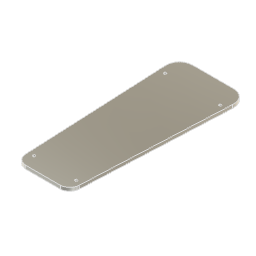
mission_engineering_pr1_pedal_raiser_kit v1 (Autodesk Fusion 360 design; units mm, degrees)
Autodesk Fusion 360 part; units mm, degrees
sketch "Sketch2" plane through (0, 0, 0) normal (0, 0, 1) x (1, 0, 0)
  line L0 (-41, 95) -> (40.1, 95) construction
  circle A0 centre (-41, 95) radius 1.75
  circle A1 centre (40.1, 95) radius 1.75
  line L1 (-32.1418, -106.2761) -> (29.9104, -106.2761) construction
  circle A2 centre (-32.1418, -106.2761) radius 1.75
  circle A3 centre (29.9104, -106.2761) radius 1.75
  line L2 (0, 125.7) -> (-30.2729, 125.7)
  line L3 (0, -124.4) -> (-26.7617, -124.4)
  line L4 (-40.5, -110.5) -> (-50.5, 104.7)
  arc A4 (-40.5, -110.5) -> (-26.7617, -124.4) centre (-25.9132, -109.8222) ccw
  arc A5 (-45.3008, 119.9335) -> (-50.5, 104.7) centre (-28.5694, 105.7191) ccw
  arc A6 (-30.2729, 125.7) -> (-45.3008, 119.9335) centre (-30.2729, 103.2348) ccw
  arc A7 (43.3008, 119.9335) -> (28.2729, 125.7) centre (28.2729, 103.2348) ccw
  arc A8 (48.5, 104.7) -> (43.3008, 119.9335) centre (26.5694, 105.7191) ccw
  line L5 (38.5, -110.5) -> (48.5, 104.7)
  arc A9 (24.7617, -124.4) -> (38.5, -110.5) centre (23.9132, -109.8222) ccw
  line L6 (0, 125.7) -> (28.2729, 125.7)
  line L7 (0, -124.4) -> (24.7617, -124.4)
  circle A10 centre (-41, 95) radius 3.75
  circle A11 centre (-41, 95) radius 3.75
  circle A12 centre (40.1, 95) radius 3.75
  circle A13 centre (-32.1418, -106.2761) radius 3.75
  circle A14 centre (29.9104, -106.2761) radius 3.75
  dimension "d1" = 3.5
  dimension "d2" = 62.0522
  dimension "d3" = 7.5
  dimension "d4" = 7.5
  constraint coincident L0.start A0.centre
  constraint coincident L0.end A1.centre
  constraint equal A0 A1
  constraint horizontal L1
  constraint coincident L1.start A2.centre
  constraint coincident L1.end A3.centre
  constraint equal A0 A2
  constraint equal A0 A3
  constraint tangent L4 A4
  constraint tangent L4 A5
  constraint tangent L2 A6
  constraint tangent A7 L6
  constraint parallel L3 L7
  constraint concentric A0 A10
  constraint concentric A1 A12
  constraint concentric A2 A13
  constraint concentric A3 A14
  constraint equal A10 A12
  constraint equal A10 A13
  constraint equal A10 A14
  measures "d1" diameter of A0
  measures "d2" distance of L1.start L1.end
  measures "d3" diameter of A10
  measures "d4" diameter of A11
extrude "Extrude1" add sketch "Sketch2" along normal blind 5 contours L2 L3 L4 A4 A5 A6 A7 A8 L5 A9 L6 L7 | A10 A11 | A12 | A13 | A14
extrude "Extrude2" cut sketch "Sketch2" along normal blind 2.5 contours A10 A11 | A12 | A13 | A14
